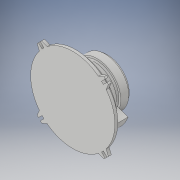
# Autodesk Inventor part: speaker
Saved by Autodesk Inventor 2017 (Build 210142000, 142)
## iProperties
Created: 2018-07-22
Part Number: speaker
Material: Generic
Document SubType Name: Modeling
Designer: Jake
Density: 1 g/cm^3
Appearance: Default
Author: Jake
Autodesk Inventor part; units mm, degrees
ref_plane "YZ Plane" through (0, 0, 0) normal (1, 0, 0) x (0, 1, 0)
ref_plane "XZ Plane" through (0, 0, 0) normal (0, 1, 0) x (-1, 0, 0)
sketch "Sketch1" plane through (0, 0, 0) normal (0, 0, 1) x (1, 0, 0)
  circle A0 centre (0, 0) radius 45
  dimension "d0" = 90
  constraints: 1 centre point, 1 coincident
  measures "d0" diameter of A0
extrude "Extrusion1" add sketch "Sketch1" along normal blind 15
sketch "Sketch2" plane through (0, 0, 0) normal (0, 0, -1) x (-1, 0, 0)
  circle A0 centre (0, 0) radius 41.5
  dimension "d3" = 83
  constraints: 1 centre point, 1 coincident
  measures "d3" diameter of A0
extrude "Extrusion2" add sketch "Sketch2" along normal blind 4.5
sketch "Sketch3" plane through (0, 0, 15) normal (0, 0, 1) x (1, 0, 0)
  circle A0 centre (0, 0) radius 41.5
  circle A1 centre (0, 0) radius 41.5 projected
  constraints: 2 concentric, 1 centre point, 1 coincident
extrude "Extrusion3" add sketch "Sketch3" along normal blind 4.5
ref_plane "Work Plane1" through (0, 0, 55) normal (0, 0, -1) x (-1, 0, 0)
sketch "Sketch4" plane through (0, 0, 55) normal (0, 0, -1) x (-1, 0, 0)
  circle A0 centre (0, 0) radius 69.5
  dimension "d9" = 139
  constraints: 1 centre point, 1 coincident
  measures "d9" diameter of A0
extrude "Extrusion4" add sketch "Sketch4" along normal blind 8.5
loft "Loft1" add section 1 edges at (69.5, 0, 46.5) section 2 edges at (-41.5, 0, 19.5)
sketch "Sketch5" plane through (0, 0, 15) normal (0, 0, 1) x (1, 0, 0)
  circle A0 centre (0, 0) radius 69.5 projected
  circle A1 centre (0, 0) radius 41.5 projected
  circle A2 centre (0, 0) radius 41.5 projected
  arc A3 (-40.1742, -47.8778) -> (58.7308, -21.3763) centre (0, 0) ccw
  line L0 (58.7308, -21.3763) -> (38.9972, -14.1938)
  circle A4 centre (0, 0) radius 41.5 projected
  line L1 (-40.1742, -47.8778) -> (-26.6757, -31.7908)
  line L2 (0, 0) -> (24.5458, 0) construction
  dimension "d16" = 21
  dimension "d17" = 20
  dimension "d18" = 50
  constraints: 6 end point, 6 point on circle, 2 line through centre, 1 centre point, 1 concentric, 1 horizontal
  measures "d16" radial gap between concentric circles of A3 A1
  measures "d17" angle of L0 L2
  measures "d18" angle of L1 L2
extrude "Extrusion5" add sketch "Sketch5" along normal blind 20.5 contours A1 L0 A3 L1
sketch "Sketch6" plane through (0, 0, 55) normal (0, 0, 1) x (1, 0, 0)
  circle A0 centre (0, 0) radius 79.375
  dimension "d21" = 158.75
  constraints: 1 centre point, 1 coincident
  measures "d21" diameter of A0
extrude "Extrusion6" add sketch "Sketch6" along normal blind 5.5
sketch "Sketch7" plane through (0, 0, 60.5) normal (0, 0, 1) x (1, 0, 0)
  circle A0 centre (0, 0) radius 79.375 projected
  line L0 (-90.0773, 90.0773) -> (90.0773, -90.0773)
  line L1 (93.9163, 93.9163) -> (-93.9163, -93.9163)
  line L2 (0, 101.3033) -> (0, -101.3033)
  line L3 (-62.9282, 62.9282) -> (-55.15, 55.15) construction
  line L4 (-64.6959, 61.1604) -> (-56.9178, 53.3822)
  line L5 (-53.3822, 56.9178) -> (-61.1604, 64.6959)
  arc A1 (-61.1604, 64.6959) -> (-64.6959, 61.1604) centre (-62.9282, 62.9282) ccw
  arc A2 (-56.9178, 53.3822) -> (-53.3822, 56.9178) centre (-55.15, 55.15) ccw
  line L6 (62.9282, 62.9282) -> (55.15, 55.15) construction
  line L7 (61.1604, 64.6959) -> (53.3822, 56.9178)
  line L8 (56.9178, 53.3822) -> (64.6959, 61.1604)
  arc A3 (64.6959, 61.1604) -> (61.1604, 64.6959) centre (62.9282, 62.9282) ccw
  arc A4 (53.3822, 56.9178) -> (56.9178, 53.3822) centre (55.15, 55.15) ccw
  line L9 (-55.15, -55.15) -> (-62.9282, -62.9282) construction
  line L10 (-56.9178, -53.3822) -> (-64.6959, -61.1604)
  line L11 (-61.1604, -64.6959) -> (-53.3822, -56.9178)
  arc A5 (-53.3822, -56.9178) -> (-56.9178, -53.3822) centre (-55.15, -55.15) ccw
  arc A6 (-64.6959, -61.1604) -> (-61.1604, -64.6959) centre (-62.9282, -62.9282) ccw
  line L12 (55.15, -55.15) -> (62.9282, -62.9282) construction
  line L13 (53.3822, -56.9178) -> (61.1604, -64.6959)
  line L14 (64.6959, -61.1604) -> (56.9178, -53.3822)
  arc A7 (56.9178, -53.3822) -> (53.3822, -56.9178) centre (55.15, -55.15) ccw
  arc A8 (61.1604, -64.6959) -> (64.6959, -61.1604) centre (62.9282, -62.9282) ccw
  line L15 (-61.1604, 64.6959) -> (-58.6855, 67.1708)
  line L16 (-58.6855, 67.1708) -> (-48.3688, 62.9352)
  circle A9 centre (0, 0) radius 79.375 projected
  line L17 (-64.6959, 61.1604) -> (-67.1708, 58.6855)
  line L18 (-67.1708, 58.6855) -> (-62.9352, 48.3688)
  line L19 (64.6959, 61.1604) -> (67.1708, 58.6855)
  line L20 (67.1708, 58.6855) -> (62.9352, 48.3688)
  line L21 (61.1604, 64.6959) -> (58.6855, 67.1708)
  line L22 (58.6855, 67.1708) -> (48.3688, 62.9352)
  line L23 (64.6959, -61.1604) -> (67.1708, -58.6855)
  line L24 (67.1708, -58.6855) -> (62.9352, -48.3688)
  line L25 (61.1604, -64.6959) -> (58.6855, -67.1708)
  line L26 (58.6855, -67.1708) -> (48.3688, -62.9352)
  line L27 (-61.1604, -64.6959) -> (-58.6855, -67.1708)
  line L28 (-58.6855, -67.1708) -> (-48.3688, -62.9352)
  line L29 (-64.6959, -61.1604) -> (-67.1708, -58.6855)
  line L30 (-67.1708, -58.6855) -> (-62.9352, -48.3688)
  point P0 (-59.0391, 59.0391)
  point P1 (59.0391, 59.0391)
  point P2 (-59.0391, -59.0391)
  point P3 (59.0391, -59.0391)
  dimension "d24" = 45
  dimension "d25" = 45
  dimension "d26" = 5
  dimension "d27" = 5
  dimension "d28" = 11
  dimension "d29" = 11
  dimension "d30" = 110.3
  dimension "d31" = 5
  dimension "d32" = 5
  dimension "d33" = 11
  dimension "d34" = 11
  dimension "d35" = 110.3
  dimension "d36" = 3.5
  dimension "d37" = 7.8
  dimension "d38" = 3.5
  dimension "d39" = 7.8
  dimension "d40" = 3.5
  dimension "d41" = 3.5
  dimension "d42" = 7.8
  dimension "d43" = 7.8
  dimension "d44" = 3.5
  dimension "d45" = 3.5
  dimension "d46" = 7.8
  dimension "d47" = 7.8
  dimension "d48" = 3.5
  dimension "d49" = 3.5
  dimension "d50" = 7.8
  dimension "d51" = 7.8
  constraints: 70 end point, 16 point on circle, 16 tangent, 11 point on line, 8 centre point, 7 midpoint, 5 perpendicular, 4 parallel, 2 horizontal alignment, 1 coincident, 1 vertical, 18 other
  measures "d24" angle of L2 L1
  measures "d25" angle of L2 L0
  measures "d26" diameter of A2
  measures "d27" diameter of A4
  measures "d28" distance of L3.end L3.start
  measures "d29" distance of L6.end L6.start
  measures "d30" distance of L6.end L3.end
  measures "d31" diameter of A6
  measures "d32" diameter of A8
  measures "d33" distance of L9.start L9.end
  measures "d34" distance of L12.start L12.end
  measures "d35" distance of L12.start L9.start
  measures "d36" distance of L5.end L15.end
  measures "d37" distance from line of L5 L16.end
  measures "d38" distance of L4.start L17.end
  measures "d39" distance from line of L4 L18.end
  measures "d40" distance of L7.start L21.end
  measures "d41" distance of L8.end L19.end
  measures "d42" distance from line of L7 L22.end
  measures "d43" distance from line of L8 L20.end
  measures "d44" distance of L14.start L23.end
  measures "d45" distance of L13.end L25.end
  measures "d46" distance from line of L14 L24.end
  measures "d47" distance from line of L13 L26.end
  measures "d48" distance of L11.start L27.end
  measures "d49" distance of L10.end L29.end
  measures "d50" distance from line of L11 L28.end
  measures "d51" distance from line of L10 L30.end
extrude "Extrusion7" add sketch "Sketch7" against normal up to surface (5.5 mm away) contours A0 L14 A7 L0 L1 A4 L8 | A0 L8 L19 L20 | L24 L23 L14 A0 | L8 A4 L1 A0 | A0 L0 A7 L14 | L1 A4 L7 A0 | A0 L13 A7 L0 | L7 A4 L1 L2 A0 | A0 L22 L21 L7 | L13 L25 L26 A0 | A0 L2 L0 A7 L13 | L1 A5 L10 A0 L4 A2 L0 | L2 A0 L11 A5 L1 | L0 A2 L5 A0 L2 | A2 L4 A0 L0 | L0 A0 L5 A2 | A5 L11 A0 L1 | L1 A0 L10 A5 | A0 L5 L15 L16 | L28 L27 L11 A0 | A0 L18 L17 L4 | L10 L29 L30 A0
sketch "Sketch9" plane through (0, 0, 0) normal (0, 0, -1) x (-1, 0, 0)
  arc A0 (28.9254, -34.472) -> (-42.2862, -15.3909) centre (0, 0) ccw projected
  line L0 (45, 3.175) -> (51.35, 3.175)
  line L1 (51.35, 3.175) -> (51.35, -3.175)
  line L2 (51.35, -3.175) -> (45, -3.175)
  line L3 (45, -3.175) -> (45, 3.175)
  point P0 (45, 0)
  dimension "d54" = 6.35
  dimension "d55" = 6.35
  constraints: 8 end point, 2 parallel, 1 horizontal, 1 horizontal alignment, 1 midpoint, 1 perpendicular, 1 tangent
  measures "d54" distance between parallel lines of L2 L0
  measures "d55" distance of L0.start L0.end
extrude "Extrusion8" add sketch "Sketch9" against normal blind 6.35
equation "\"d29\" = d28"
equation "\"d33\" = d28"
equation "\"d34\" = d28"
equation "\"d35\" = d30"
equation "\"d38\" = d36"
equation "\"d39\" = d37"
equation "\"d40\" = d36"
equation "\"d41\" = d40"
equation "\"d42\" = d37"
equation "\"d43\" = d42"
equation "\"d44\" = d36"
equation "\"d45\" = d44"
equation "\"d46\" = d37"
equation "\"d47\" = d46"
equation "\"d48\" = d36"
equation "\"d49\" = d48"
equation "\"d50\" = d39"
equation "\"d51\" = d50"
equation "\"d55\" = d54"
body "Solid1"
